Autodesk Inventor part; units mm, degrees
(part 5 of 6)
  line L796 (-0.8981, -221.2353) -> (-1.2073, -221.1704) construction
  line L797 (-1.2073, -221.1704) -> (-1.274, -221.1564) construction
  line L798 (-1.274, -221.1564) -> (-1.3926, -221.1187) construction
  line L799 (-1.3926, -221.1187) -> (-1.5231, -221.0797) construction
  line L800 (5.0298, -224.2577) -> (4.9095, -225.6862) construction
  spline S57 degree 3 poles (5.254, -220.972) (5.1998, -222.0685) (5.122, -223.1637) (5.0298, -224.2577) (4.9095, -225.6862) (4.7534, -227.1125) (4.551, -228.5318) (4.3466, -229.9645) (4.0271, -231.4371) (4.0386, -232.8878) (4.0462, -233.8475) (5.2747, -233.8855) (5.6006, -233.0992) (6.3871, -231.2018) (6.5459, -228.982) (6.7906, -226.9594) (7.0368, -224.9246) (7.1993, -222.8825) (7.2738, -220.8341) (7.2885, -220.4289) (7.3025, -220.0233) (7.3103, -219.6178) knots 5.14687 5.14687 5.14687 5.14687 6 6 6 7 7 7 8 8 8 9 9 9 10 10 10 11 11 11 11.773986 11.773986 11.773986 11.773986
  line L801 (5.254, -220.972) -> (5.1998, -222.0685) construction
  line L802 (5.1998, -222.0685) -> (5.122, -223.1637) construction
  line L803 (5.122, -223.1637) -> (5.0298, -224.2577) construction
  line L804 (4.9095, -225.6862) -> (4.7534, -227.1125) construction
  line L805 (4.7534, -227.1125) -> (4.551, -228.5318) construction
  line L806 (4.551, -228.5318) -> (4.3466, -229.9645) construction
  line L807 (4.3466, -229.9645) -> (4.0271, -231.4371) construction
  line L808 (4.0271, -231.4371) -> (4.0386, -232.8878) construction
  line L809 (4.0386, -232.8878) -> (4.0462, -233.8475) construction
  line L810 (4.0462, -233.8475) -> (5.2747, -233.8855) construction
  line L811 (5.2747, -233.8855) -> (5.6006, -233.0992) construction
  line L812 (5.6006, -233.0992) -> (6.3871, -231.2018) construction
  line L813 (6.3871, -231.2018) -> (6.5459, -228.982) construction
  line L814 (6.5459, -228.982) -> (6.7906, -226.9594) construction
  line L815 (6.7906, -226.9594) -> (7.0368, -224.9246) construction
  line L816 (7.0368, -224.9246) -> (7.1993, -222.8825) construction
  line L817 (7.1993, -222.8825) -> (7.2738, -220.8341) construction
  line L818 (7.2738, -220.8341) -> (7.2885, -220.4289) construction
  line L819 (7.2885, -220.4289) -> (7.3025, -220.0233) construction
  line L820 (7.3025, -220.0233) -> (7.3103, -219.6178) construction
  line L821 (-2.0297, -225.1684) -> (-2.0388, -225.06) construction
  spline S58 degree 3 poles (-2.0297, -225.1684) (-2.0388, -225.06) (-2.0694, -224.9045) (-2.0732, -224.8323) knots 8.458233 8.458233 8.458233 8.458233 9 9 9 9
  line L822 (-2.0388, -225.06) -> (-2.0694, -224.9045) construction
  line L823 (-2.0694, -224.9045) -> (-2.0732, -224.8323) construction
  line L824 (-2.0856, -224.5997) -> (-2.0972, -224.3671) construction
  spline S59 degree 3 poles (-2.0732, -224.8323) (-2.0856, -224.5997) (-2.0972, -224.3671) (-2.109, -224.1346) knots 9 9 9 9 10 10 10 10
  line L825 (-2.0732, -224.8323) -> (-2.0856, -224.5997) construction
  line L826 (-2.0972, -224.3671) -> (-2.109, -224.1346) construction
  line L827 (-1.5231, -221.0797) -> (-1.328, -220.9404) construction
  spline S60 degree 3 poles (-1.5231, -221.0797) (-1.328, -220.9404) (-1.1366, -220.7956) (-0.9498, -220.6454) (-0.1242, -219.9816) (0.9816, -219.0458) (1.2926, -217.9913) (2.0159, -215.5393) (-1.1884, -215.1481) (-2.8267, -215.345) (-5.2805, -215.6397) (-7.7108, -216.8198) (-9.2996, -218.7397) (-9.8909, -219.4541) (-8.9514, -220.4463) (-8.2639, -219.7754) knots 21.261625 21.261625 21.261625 21.261625 22 22 22 23 23 23 24 24 24 25 25 25 26 26 26 26
  line L828 (-1.328, -220.9404) -> (-1.1366, -220.7956) construction
  line L829 (-1.1366, -220.7956) -> (-0.9498, -220.6454) construction
  line L830 (-0.9498, -220.6454) -> (-0.1242, -219.9816) construction
  line L831 (-0.1242, -219.9816) -> (0.9816, -219.0458) construction
  line L832 (0.9816, -219.0458) -> (1.2926, -217.9913) construction
  line L833 (1.2926, -217.9913) -> (2.0159, -215.5393) construction
  line L834 (2.0159, -215.5393) -> (-1.1884, -215.1481) construction
  line L835 (-1.1884, -215.1481) -> (-2.8267, -215.345) construction
  line L836 (-2.8267, -215.345) -> (-5.2805, -215.6397) construction
  line L837 (-5.2805, -215.6397) -> (-7.7108, -216.8198) construction
  line L838 (-7.7108, -216.8198) -> (-9.2996, -218.7397) construction
  line L839 (-9.2996, -218.7397) -> (-9.8909, -219.4541) construction
  line L840 (-9.8909, -219.4541) -> (-8.9514, -220.4463) construction
  line L841 (-8.9514, -220.4463) -> (-8.2639, -219.7754) construction
  line L842 (-2.1476, -223.2875) -> (-2.1533, -222.8634) construction
  spline S61 degree 3 poles (-2.109, -224.1346) (-2.1305, -223.7108) (-2.1476, -223.2875) (-2.1533, -222.8634) knots 10 10 10 10 10.82684 10.82684 10.82684 10.82684
  line L843 (-2.109, -224.1346) -> (-2.1305, -223.7108) construction
  line L844 (-2.1305, -223.7108) -> (-2.1476, -223.2875) construction
  line L845 (4.252, -221.2799) -> (5.254, -220.972) construction
  spline S62 degree 3 poles (2.1677, -216.0966) (0.6747, -217.2243) (0.7113, -219.4286) (2.2363, -220.5301) (3.1577, -221.1955) (4.252, -221.2799) (5.254, -220.972) knots 0 0 0 0 1 1 1 1.551759 1.551759 1.551759 1.551759
  line L846 (2.1677, -216.0966) -> (0.6747, -217.2243) construction
  line L847 (0.6747, -217.2243) -> (0.7113, -219.4286) construction
  line L848 (0.7113, -219.4286) -> (2.2363, -220.5301) construction
  line L849 (2.2363, -220.5301) -> (3.1577, -221.1955) construction
  line L850 (3.1577, -221.1955) -> (4.252, -221.2799) construction
  line L851 (7.3103, -219.6178) -> (7.3306, -219.5942) construction
  spline S63 degree 3 poles (7.3103, -219.6178) (7.3306, -219.5942) (7.3507, -219.5703) (7.3705, -219.5463) (7.9707, -218.8184) (8.5772, -217.7782) (7.9557, -216.8786) (7.3563, -216.011) (6.1286, -216.1196) (5.6288, -217.0177) (5.3108, -217.589) (5.2677, -218.349) (5.2721, -219.0878) knots 1.983848 1.983848 1.983848 1.983848 2 2 2 3 3 3 4 4 4 4.613609 4.613609 4.613609 4.613609
  line L852 (7.3306, -219.5942) -> (7.3507, -219.5703) construction
  line L853 (7.3507, -219.5703) -> (7.3705, -219.5463) construction
  line L854 (7.3705, -219.5463) -> (7.9707, -218.8184) construction
  line L855 (7.9707, -218.8184) -> (8.5772, -217.7782) construction
  line L856 (8.5772, -217.7782) -> (7.9557, -216.8786) construction
  line L857 (7.9557, -216.8786) -> (7.3563, -216.011) construction
  line L858 (7.3563, -216.011) -> (6.1286, -216.1196) construction
  line L859 (6.1286, -216.1196) -> (5.6288, -217.0177) construction
  line L860 (5.6288, -217.0177) -> (5.3108, -217.589) construction
  line L861 (5.3108, -217.589) -> (5.2677, -218.349) construction
  line L862 (5.2677, -218.349) -> (5.2721, -219.0878) construction
  line L863 (5.2721, -219.0878) -> (5.1898, -219.1386) construction
  spline S64 degree 3 poles (5.2721, -219.0878) (5.1898, -219.1386) (5.1044, -219.1847) (5.0157, -219.2254) (4.3643, -219.5238) (3.4605, -219.4778) (2.9536, -218.9221) (2.5045, -218.4298) (2.5751, -217.6746) (3.0552, -217.2469) (3.6655, -216.7032) (2.837, -215.591) (2.1677, -216.0966) knots 16.74527 16.74527 16.74527 16.74527 17 17 17 18 18 18 19 19 19 20 20 20 20
  line L864 (5.1898, -219.1386) -> (5.1044, -219.1847) construction
  line L865 (5.1044, -219.1847) -> (5.0157, -219.2254) construction
  line L866 (5.0157, -219.2254) -> (4.3643, -219.5238) construction
  line L867 (4.3643, -219.5238) -> (3.4605, -219.4778) construction
  line L868 (3.4605, -219.4778) -> (2.9536, -218.9221) construction
  line L869 (2.9536, -218.9221) -> (2.5045, -218.4298) construction
  line L870 (2.5045, -218.4298) -> (2.5751, -217.6746) construction
  line L871 (2.5751, -217.6746) -> (3.0552, -217.2469) construction
  line L872 (3.0552, -217.2469) -> (3.6655, -216.7032) construction
  line L873 (3.6655, -216.7032) -> (2.837, -215.591) construction
  line L874 (2.837, -215.591) -> (2.1677, -216.0966) construction
  circle A5 centre (6.8365, -217.7782) radius 0.6286
  line L875 (-1.4966, -218.9144) -> (-2.1126, -219.3576) construction
  spline S65 degree 3 poles (-8.2639, -219.7754) (-6.7861, -218.3333) (-5.0043, -217.3238) (-2.9422, -217.0238) (-2.3715, -216.9407) (-0.7769, -216.6798) (-0.3673, -217.2886) (-0.0416, -217.7728) (-1.4966, -218.9144) (-2.1126, -219.3576) knots 0 0 0 0 1 1 1 2 2 2 2.88117 2.88117 2.88117 2.88117
  line L876 (-8.2639, -219.7754) -> (-6.7861, -218.3333) construction
  line L877 (-6.7861, -218.3333) -> (-5.0043, -217.3238) construction
  line L878 (-5.0043, -217.3238) -> (-2.9422, -217.0238) construction
  line L879 (-2.9422, -217.0238) -> (-2.3715, -216.9407) construction
  line L880 (-2.3715, -216.9407) -> (-0.7769, -216.6798) construction
  line L881 (-0.7769, -216.6798) -> (-0.3673, -217.2886) construction
  line L882 (-0.3673, -217.2886) -> (-0.0416, -217.7728) construction
  line L883 (-0.0416, -217.7728) -> (-1.4966, -218.9144) construction
  point P0 (0, 0)
  point P1 (-89.8672, -198.2095)
  point P2 (-69.9742, -200.3683)
  point P3 (-75.8668, -170.3202)
  point P4 (-42.8129, -214.4515)
  point P5 (-41.2254, -216.039)
  point P6 (-53.6547, -194.1688)
  point P7 (-90.9293, -176.9978)
  point P8 (-2.0909, -219.5286)
  constraints: 6 centre point, 180 other
extrude "Extrusion5" add sketch "Sketch6" against normal up to surface (3.175 mm away)
sketch "Sketch7" plane through (0, 3.175, 0) normal (0, 1, 0) x (1, 0, 0)
  circle A0 centre (16.8645, 29.5775) radius 1.25 projected
  circle A1 centre (-15.1355, 29.5775) radius 1.25 projected
  circle A2 centre (-15.1355, 61.5775) radius 1.25 projected
  circle A3 centre (16.8645, 61.5775) radius 1.25 projected
  arc A4 (15.8645, 52.5775) -> (15.8645, 54.5775) centre (15.8645, 53.5775) ccw projected
  line L0 (15.8645, 52.5775) -> (-23.218, 52.5775) projected
  arc A5 (-23.218, 52.5775) -> (-23.218, 50.5775) centre (-23.218, 51.5775) ccw projected
  line L1 (-23.218, 50.5775) -> (15.8645, 50.5775) projected
  arc A6 (15.8645, 48.5775) -> (15.8645, 50.5775) centre (15.8645, 49.5775) ccw projected
  line L2 (15.8645, 48.5775) -> (-23.218, 48.5775) projected
  arc A7 (-23.218, 48.5775) -> (-23.218, 46.5775) centre (-23.218, 47.5775) ccw projected
  line L3 (-23.218, 46.5775) -> (15.8645, 46.5775) projected
  arc A8 (15.8645, 44.5775) -> (15.8645, 46.5775) centre (15.8645, 45.5775) ccw projected
  line L4 (15.8645, 44.5775) -> (-23.218, 44.5775) projected
  arc A9 (-23.218, 44.5775) -> (-23.218, 42.5775) centre (-23.218, 43.5775) ccw projected
  line L5 (-23.218, 42.5775) -> (15.8645, 42.5775) projected
  arc A10 (15.8645, 40.5775) -> (15.8645, 42.5775) centre (15.8645, 41.5775) ccw projected
  line L6 (15.8645, 40.5775) -> (-23.218, 40.5775) projected
  arc A11 (-23.218, 40.5775) -> (-23.218, 38.5775) centre (-23.218, 39.5775) ccw projected
  line L7 (-23.218, 38.5775) -> (15.8645, 38.5775) projected
  arc A12 (15.8645, 36.5775) -> (15.8645, 38.5775) centre (15.8645, 37.5775) ccw projected
  line L8 (15.8645, 36.5775) -> (-23.218, 36.5775) projected
  arc A13 (-23.218, 36.5775) -> (-23.218, 34.5775) centre (-23.218, 35.5775) ccw projected
  line L9 (-23.218, 34.5775) -> (15.8645, 34.5775) projected
  arc A14 (15.8645, 32.5775) -> (15.8645, 34.5775) centre (15.8645, 33.5775) ccw projected
  line L10 (15.8645, 32.5775) -> (-21.0398, 32.5775) projected
  arc A15 (-21.0398, 32.5775) -> (-26.4124, 32.0925) centre (-21.0398, 2.5775) ccw projected
  arc A16 (-31.785, 31.6075) -> (-26.4124, 32.0925) centre (-31.785, 61.6075) ccw projected
  line L11 (-31.785, 31.6075) -> (-33.743, 31.6075) projected
  arc A17 (-33.743, 31.6075) -> (-40.093, 25.2575) centre (-33.743, 25.2575) ccw projected
  line L12 (-40.093, 25.2575) -> (-40.093, 19.225) projected
  arc A18 (-40.093, 19.225) -> (-38.5055, 17.6375) centre (-38.5055, 19.225) ccw projected
  line L13 (-38.5055, 17.6375) -> (36.4245, 17.6375) projected
  arc A19 (36.4245, 17.6375) -> (38.012, 19.225) centre (36.4245, 19.225) ccw projected
  line L14 (38.012, 19.225) -> (38.012, 71.9264) projected
  arc A20 (38.012, 71.9264) -> (36.4245, 73.5139) centre (36.4245, 71.9264) ccw projected
  line L15 (36.4245, 73.5139) -> (-37.8705, 73.5139) projected
  arc A21 (-37.8705, 73.5139) -> (-39.458, 71.9264) centre (-37.8705, 71.9264) ccw projected
  line L16 (-39.458, 71.9264) -> (-39.458, 65.8975) projected
  arc A22 (-39.458, 65.8975) -> (-33.108, 59.5475) centre (-33.108, 65.8975) ccw projected
  line L17 (-33.108, 59.5475) -> (-31.785, 59.5475) projected
  arc A23 (-26.4124, 59.0625) -> (-31.785, 59.5475) centre (-31.785, 29.5475) ccw projected
  arc A24 (-26.4124, 59.0625) -> (-21.0398, 58.5775) centre (-21.0398, 88.5775) ccw projected
  line L18 (-21.0398, 58.5775) -> (15.8645, 58.5775) projected
  arc A25 (15.8645, 56.5775) -> (15.8645, 58.5775) centre (15.8645, 57.5775) ccw projected
  line L19 (15.8645, 56.5775) -> (-23.218, 56.5775) projected
  arc A26 (-23.218, 56.5775) -> (-23.218, 54.5775) centre (-23.218, 55.5775) ccw projected
  line L20 (-23.218, 54.5775) -> (15.8645, 54.5775) projected
  circle A27 centre (16.6963, -6.4758) radius 1.25 projected
  circle A28 centre (-15.3037, -38.4758) radius 1.25 projected
  circle A29 centre (-15.3037, -6.4758) radius 1.25 projected
  circle A30 centre (16.6963, -38.4758) radius 1.25 projected
  line L21 (-33.2762, -8.5058) -> (-31.9532, -8.5058) projected
  arc A31 (-26.5806, -8.9908) -> (-31.9532, -8.5058) centre (-31.9532, -38.5058) ccw projected
  arc A32 (-26.5806, -8.9908) -> (-21.208, -9.4758) centre (-21.208, 20.5242) ccw projected
  line L22 (-21.208, -9.4758) -> (15.6963, -9.4758) projected
  arc A33 (15.6963, -11.4758) -> (15.6963, -9.4758) centre (15.6963, -10.4758) ccw projected
  line L23 (15.6963, -11.4758) -> (-23.3862, -11.4758) projected
  arc A34 (-23.3862, -11.4758) -> (-23.3862, -13.4758) centre (-23.3862, -12.4758) ccw projected
  line L24 (-23.3862, -13.4758) -> (15.6963, -13.4758) projected
  arc A35 (15.6963, -15.4758) -> (15.6963, -13.4758) centre (15.6963, -14.4758) ccw projected
  line L25 (15.6963, -15.4758) -> (-23.3862, -15.4758) projected
  arc A36 (-23.3862, -15.4758) -> (-23.3862, -17.4758) centre (-23.3862, -16.4758) ccw projected
  line L26 (-23.3862, -17.4758) -> (15.6963, -17.4758) projected
  arc A37 (15.6963, -19.4758) -> (15.6963, -17.4758) centre (15.6963, -18.4758) ccw projected
  line L27 (15.6963, -19.4758) -> (-23.3862, -19.4758) projected
  arc A38 (-23.3862, -19.4758) -> (-23.3862, -21.4758) centre (-23.3862, -20.4758) ccw projected
  line L28 (-23.3862, -21.4758) -> (15.6963, -21.4758) projected
  arc A39 (15.6963, -23.4758) -> (15.6963, -21.4758) centre (15.6963, -22.4758) ccw projected
  line L29 (15.6963, -23.4758) -> (-23.3862, -23.4758) projected
  arc A40 (-23.3862, -23.4758) -> (-23.3862, -25.4758) centre (-23.3862, -24.4758) ccw projected
  line L30 (-23.3862, -25.4758) -> (15.6963, -25.4758) projected
  arc A41 (15.6963, -27.4758) -> (15.6963, -25.4758) centre (15.6963, -26.4758) ccw projected
  line L31 (15.6963, -27.4758) -> (-23.3862, -27.4758) projected
  arc A42 (-23.3862, -27.4758) -> (-23.3862, -29.4758) centre (-23.3862, -28.4758) ccw projected
  line L32 (-23.3862, -29.4758) -> (15.6963, -29.4758) projected
  arc A43 (15.6963, -31.4758) -> (15.6963, -29.4758) centre (15.6963, -30.4758) ccw projected
  line L33 (15.6963, -31.4758) -> (-23.3862, -31.4758) projected
  arc A44 (-23.3862, -31.4758) -> (-23.3862, -33.4758) centre (-23.3862, -32.4758) ccw projected
  line L34 (-23.3862, -33.4758) -> (15.6963, -33.4758) projected
  arc A45 (15.6963, -35.4758) -> (15.6963, -33.4758) centre (15.6963, -34.4758) ccw projected
  line L35 (15.6963, -35.4758) -> (-21.208, -35.4758) projected
  arc A46 (-21.208, -35.4758) -> (-26.5806, -35.9608) centre (-21.208, -65.4758) ccw projected
  arc A47 (-31.9532, -36.4458) -> (-26.5806, -35.9608) centre (-31.9532, -6.4458) ccw projected
  line L36 (-31.9532, -36.4458) -> (-33.9112, -36.4458) projected
  arc A48 (-33.9112, -36.4458) -> (-40.2612, -42.7958) centre (-33.9112, -42.7958) ccw projected
  line L37 (-40.2612, -42.7958) -> (-40.2612, -48.8283) projected
  arc A49 (-40.2612, -48.8283) -> (-38.6737, -50.4158) centre (-38.6737, -48.8283) ccw projected
  line L38 (-38.6737, -50.4158) -> (36.2563, -50.4158) projected
  arc A50 (36.2563, -50.4158) -> (37.8438, -48.8283) centre (36.2563, -48.8283) ccw projected
  line L39 (37.8438, -48.8283) -> (37.8438, 3.8731) projected
  arc A51 (37.8438, 3.8731) -> (36.2563, 5.4606) centre (36.2563, 3.8731) ccw projected
  line L40 (36.2563, 5.4606) -> (-38.0387, 5.4606) projected
  arc A52 (-38.0387, 5.4606) -> (-39.6262, 3.8731) centre (-38.0387, 3.8731) ccw projected
  line L41 (-39.6262, 3.8731) -> (-39.6262, -2.1558) projected
  arc A53 (-39.6262, -2.1558) -> (-33.2762, -8.5058) centre (-33.2762, -2.1558) ccw projected
  line L42 (48.3343, -57.616) -> (-46.3157, -57.616) projected
  arc A54 (-49.4907, -54.441) -> (-46.3157, -57.616) centre (-46.3157, -54.441) ccw projected
  line L43 (-49.4907, -54.441) -> (-49.4907, 82.209) projected
  arc A55 (-46.3157, 85.384) -> (-49.4907, 82.209) centre (-46.3157, 82.209) ccw projected
  line L44 (-46.3157, 85.384) -> (48.3343, 85.384) projected
  arc A56 (51.5093, 82.209) -> (48.3343, 85.384) centre (48.3343, 82.209) ccw projected
  line L45 (51.5093, 82.209) -> (51.5093, -54.441) projected
  arc A57 (48.3343, -57.616) -> (51.5093, -54.441) centre (48.3343, -54.441) ccw projected
  arc A58 (13.6478, -234.0466) -> (14.6363, -233.1974) centre (13.6478, -233.0466) ccw projected
  line L46 (13.6478, -234.0466) -> (-11.6292, -234.0466) projected
  arc A59 (-12.6177, -233.1974) -> (-11.6292, -234.0466) centre (-11.6292, -233.0466) ccw projected
  arc A60 (-12.9607, -228.674) -> (-12.6177, -233.1974) centre (17.0393, -228.674) ccw projected
  line L47 (-12.9607, -228.674) -> (-12.9607, -220.366) projected
  line L48 (-6.6107, -214.016) -> (8.6293, -214.016) projected
  line L49 (14.9793, -220.366) -> (14.9793, -228.674) projected
  arc A61 (14.6363, -233.1974) -> (14.9793, -228.674) centre (-15.0207, -228.674) ccw projected
  line L50 (6.0093, -246.3235) -> (6.0093, -276.3235) projected
  arc A62 (4.0093, -276.3235) -> (6.0093, -276.3235) centre (5.0093, -276.3235) ccw projected
  line L51 (4.0093, -276.3235) -> (4.0093, -245.3235) projected
  line L52 (4.0093, -245.3235) -> (5.0093, -245.3235) projected
  arc A63 (6.0093, -246.3235) -> (5.0093, -245.3235) centre (5.0093, -246.3235) ccw projected
  line L53 (8.0093, -276.3235) -> (8.0093, -246.3235) projected
  arc A64 (10.0093, -246.3235) -> (8.0093, -246.3235) centre (9.0093, -246.3235) ccw projected
  line L54 (10.0093, -246.3235) -> (10.0093, -276.3235) projected
  arc A65 (8.0093, -276.3235) -> (10.0093, -276.3235) centre (9.0093, -276.3235) ccw projected
  line L55 (0.0093, -276.3235) -> (0.0093, -246.3235) projected
  arc A66 (2.0093, -246.3235) -> (0.0093, -246.3235) centre (1.0093, -246.3235) ccw projected
  line L56 (2.0093, -246.3235) -> (2.0093, -276.3235) projected
  arc A67 (0.0093, -276.3235) -> (2.0093, -276.3235) centre (1.0093, -276.3235) ccw projected
  line L57 (-3.9907, -276.3235) -> (-3.9907, -246.3235) projected
  arc A68 (-1.9907, -246.3235) -> (-3.9907, -246.3235) centre (-2.9907, -246.3235) ccw projected
  line L58 (-1.9907, -246.3235) -> (-1.9907, -276.3235) projected
  arc A69 (-3.9907, -276.3235) -> (-1.9907, -276.3235) centre (-2.9907, -276.3235) ccw projected
  line L59 (-7.9907, -276.3235) -> (-7.9907, -246.3235) projected
  arc A70 (-5.9907, -246.3235) -> (-7.9907, -246.3235) centre (-6.9907, -246.3235) ccw projected
  line L60 (-5.9907, -246.3235) -> (-5.9907, -276.3235) projected
  arc A71 (-7.9907, -276.3235) -> (-5.9907, -276.3235) centre (-6.9907, -276.3235) ccw projected
  line L61 (-11.9907, -276.3235) -> (-11.9907, -246.3235) projected
  arc A72 (-9.9907, -246.3235) -> (-11.9907, -246.3235) centre (-10.9907, -246.3235) ccw projected
  line L62 (-9.9907, -246.3235) -> (-9.9907, -276.3235) projected
  arc A73 (-11.9907, -276.3235) -> (-9.9907, -276.3235) centre (-10.9907, -276.3235) ccw projected
  line L63 (12.0093, -276.3235) -> (12.0093, -246.3235) projected
  arc A74 (14.0093, -246.3235) -> (12.0093, -246.3235) centre (13.0093, -246.3235) ccw projected
  line L64 (14.0093, -246.3235) -> (14.0093, -276.3235) projected
  arc A75 (12.0093, -276.3235) -> (14.0093, -276.3235) centre (13.0093, -276.3235) ccw projected
  circle A76 centre (92.1343, 51.998) radius 2.5527 projected
  circle A77 centre (92.1343, 74.223) radius 2.5527 projected
  circle A78 centre (92.1343, 29.773) radius 2.5527 projected
  circle A79 centre (92.1343, -14.677) radius 2.5527 projected
  circle A80 centre (92.1343, -59.127) radius 2.5527 projected
  circle A81 centre (92.1343, -103.577) radius 2.5527 projected
  circle A82 centre (92.1343, -125.802) radius 2.5527 projected
  circle A83 centre (92.1343, -81.352) radius 2.5527 projected
  circle A84 centre (92.1343, -36.902) radius 2.5527 projected
  circle A85 centre (92.1343, 7.548) radius 2.5527 projected
  circle A86 centre (-90.1157, 51.998) radius 2.5527 projected
  circle A87 centre (-90.1157, 7.548) radius 2.5527 projected
  circle A88 centre (-90.1157, -36.902) radius 2.5527 projected
  circle A89 centre (-90.1157, -81.352) radius 2.5527 projected
  circle A90 centre (-90.1157, -125.802) radius 2.5527 projected
  circle A91 centre (-90.1157, -103.577) radius 2.5527 projected
  circle A92 centre (-90.1157, -59.127) radius 2.5527 projected
  circle A93 centre (-90.1157, -14.677) radius 2.5527 projected
  circle A94 centre (-90.1157, 29.773) radius 2.5527 projected
  circle A95 centre (-90.1157, 74.223) radius 2.5527 projected
  circle A96 centre (1.0093, 127.4103) radius 2.5527 projected
  circle A97 centre (66.2468, -142.6982) radius 2.0193 projected
  circle A98 centre (-64.2282, -31.5732) radius 2.0193 projected
  circle A99 centre (66.2468, 79.5518) radius 2.0193 projected
  circle A100 centre (66.2468, -31.5732) radius 2.0193 projected
  circle A101 centre (-64.2282, 79.5518) radius 2.0193 projected
  circle A102 centre (-64.2282, -142.6982) radius 2.0193 projected
  circle A103 centre (-4.4907, -86.566) radius 1.6 projected
  circle A104 centre (-24.9907, -156.566) radius 1.6 projected
  circle A105 centre (27.0093, -73.616) radius 1.6 projected
  circle A106 centre (59.0093, -120.616) radius 1.6 projected
  circle A107 centre (59.0093, -73.616) radius 1.6 projected
  circle A108 centre (27.0093, -120.616) radius 1.6 projected
  circle A109 centre (-45.4907, -86.566) radius 1.6 projected
  circle A110 centre (-14.9907, -277.3235) radius 1.25 projected
  circle A111 centre (17.0093, -245.3235) radius 1.25 projected
  circle A112 centre (-14.9907, -245.3235) radius 1.25 projected
  circle A113 centre (17.0093, -277.3235) radius 1.25 projected
  line L65 (-26.9307, -253.9347) -> (-26.9307, -296.8835) projected
  arc A114 (-26.9307, -296.8835) -> (-25.3432, -298.471) centre (-25.3432, -296.8835) ccw projected
  line L66 (-25.3432, -298.471) -> (27.3618, -298.471) projected
  arc A115 (27.3618, -298.471) -> (28.9493, -296.8835) centre (27.3618, -296.8835) ccw projected
  line L67 (28.9493, -296.8835) -> (28.9493, -253.9347) projected
  arc A116 (33.1552, -225.0046) -> (28.9493, -253.9347) centre (130.5493, -253.9347) ccw projected
  line L68 (70.3843, -155.8506) -> (89.4343, -144.852) projected
  line L69 (101.6593, -123.6777) -> (101.6593, 85.3463) projected
  arc A117 (101.6593, 85.3463) -> (88.4997, 104.1401) centre (81.6593, 85.3463) ccw projected
  line L70 (88.4997, 104.1401) -> (18.1103, 129.7598) projected
  arc A118 (18.1103, 129.7598) -> (-16.0917, 129.7598) centre (1.0093, 82.7751) ccw projected
  line L71 (-16.0917, 129.7598) -> (-86.4811, 104.1401) projected
  arc A119 (-86.4811, 104.1401) -> (-99.6407, 85.3463) centre (-79.6407, 85.3463) ccw projected
  line L72 (-99.6407, 85.3463) -> (-99.6407, -123.6777) projected
  line L73 (-87.4157, -144.852) -> (-68.3657, -155.8506) projected
  arc A120 (-26.9307, -253.9347) -> (-31.1366, -225.0046) centre (-128.5307, -253.9347) ccw projected
  circle A121 centre (-86.7529, -269.1865) radius 1.25 projected
  circle A122 centre (-54.7529, -269.1865) radius 1.25 projected
  circle A123 centre (-86.7529, -237.1865) radius 1.25 projected
  circle A124 centre (-54.7529, -237.1865) radius 1.25 projected
  line L74 (-44.4004, -216.039) -> (-97.1018, -216.039) projected
  arc A125 (-97.1018, -216.039) -> (-98.6893, -217.6265) centre (-97.1018, -217.6265) ccw projected
  line L75 (-98.6893, -217.6265) -> (-98.6893, -291.9215) projected
  arc A126 (-98.6893, -291.9215) -> (-97.1018, -293.509) centre (-97.1018, -291.9215) ccw projected
  line L76 (-97.1018, -293.509) -> (-91.0729, -293.509) projected
  arc A127 (-91.0729, -293.509) -> (-84.7229, -287.159) centre (-91.0729, -287.159) ccw projected
  line L77 (-84.7229, -287.159) -> (-84.7229, -285.836) projected
  arc A128 (-84.2379, -280.4634) -> (-84.7229, -285.836) centre (-54.7229, -285.836) ccw projected
  arc A129 (-84.2379, -280.4634) -> (-83.7529, -275.0908) centre (-113.7529, -275.0908) ccw projected
  line L78 (-83.7529, -275.0908) -> (-83.7529, -238.1865) projected
  arc A130 (-81.7529, -238.1865) -> (-83.7529, -238.1865) centre (-82.7529, -238.1865) ccw projected
  line L79 (-81.7529, -238.1865) -> (-81.7529, -277.269) projected
  arc A131 (-81.7529, -277.269) -> (-79.7529, -277.269) centre (-80.7529, -277.269) ccw projected
  line L80 (-79.7529, -277.269) -> (-79.7529, -238.1865) projected
  arc A132 (-77.7529, -238.1865) -> (-79.7529, -238.1865) centre (-78.7529, -238.1865) ccw projected
  line L81 (-77.7529, -238.1865) -> (-77.7529, -277.269) projected
  arc A133 (-77.7529, -277.269) -> (-75.7529, -277.269) centre (-76.7529, -277.269) ccw projected
  line L82 (-75.7529, -277.269) -> (-75.7529, -238.1865) projected
  arc A134 (-73.7529, -238.1865) -> (-75.7529, -238.1865) centre (-74.7529, -238.1865) ccw projected
  line L83 (-73.7529, -238.1865) -> (-73.7529, -277.269) projected
  arc A135 (-73.7529, -277.269) -> (-71.7529, -277.269) centre (-72.7529, -277.269) ccw projected
  line L84 (-71.7529, -277.269) -> (-71.7529, -238.1865) projected
  arc A136 (-69.7529, -238.1865) -> (-71.7529, -238.1865) centre (-70.7529, -238.1865) ccw projected
  line L85 (-69.7529, -238.1865) -> (-69.7529, -277.269) projected
  arc A137 (-69.7529, -277.269) -> (-67.7529, -277.269) centre (-68.7529, -277.269) ccw projected
  line L86 (-67.7529, -277.269) -> (-67.7529, -238.1865) projected
  arc A138 (-65.7529, -238.1865) -> (-67.7529, -238.1865) centre (-66.7529, -238.1865) ccw projected
  line L87 (-65.7529, -238.1865) -> (-65.7529, -277.269) projected
  arc A139 (-65.7529, -277.269) -> (-63.7529, -277.269) centre (-64.7529, -277.269) ccw projected
  line L88 (-63.7529, -277.269) -> (-63.7529, -238.1865) projected
  arc A140 (-61.7529, -238.1865) -> (-63.7529, -238.1865) centre (-62.7529, -238.1865) ccw projected
  line L89 (-61.7529, -238.1865) -> (-61.7529, -277.269) projected
  arc A141 (-61.7529, -277.269) -> (-59.7529, -277.269) centre (-60.7529, -277.269) ccw projected
  line L90 (-59.7529, -277.269) -> (-59.7529, -238.1865) projected
  arc A142 (-57.7529, -238.1865) -> (-59.7529, -238.1865) centre (-58.7529, -238.1865) ccw projected
  line L91 (-57.7529, -238.1865) -> (-57.7529, -275.0908) projected
  arc A143 (-57.7529, -275.0908) -> (-57.2679, -280.4634) centre (-27.7529, -275.0908) ccw projected
  arc A144 (-56.7829, -285.836) -> (-57.2679, -280.4634) centre (-86.7829, -285.836) ccw projected
  line L92 (-56.7829, -285.836) -> (-56.7829, -287.794) projected
  arc A145 (-56.7829, -287.794) -> (-50.4329, -294.144) centre (-50.4329, -287.794) ccw projected
  line L93 (-50.4329, -294.144) -> (-44.4004, -294.144) projected
  arc A146 (-44.4004, -294.144) -> (-42.8129, -292.5565) centre (-44.4004, -292.5565) ccw projected
  line L94 (-42.8129, -292.5565) -> (-42.8129, -217.6265) projected
  arc A147 (-42.8129, -217.6265) -> (-44.4004, -216.039) centre (-44.4004, -217.6265) ccw projected
  circle A148 centre (88.5764, -269.6382) radius 1.25 projected
  circle A149 centre (56.5764, -269.6382) radius 1.25 projected
  circle A150 centre (56.5764, -237.6382) radius 1.25 projected
  circle A151 centre (88.5764, -237.6382) radius 1.25 projected
  arc A152 (46.2275, -216.4907) -> (44.64, -218.0782) centre (46.2275, -218.0782) ccw projected
  line L95 (44.64, -218.0782) -> (44.64, -292.3732) projected
  arc A153 (44.64, -292.3732) -> (46.2275, -293.9607) centre (46.2275, -292.3732) ccw projected
  line L96 (46.2275, -293.9607) -> (52.2564, -293.9607) projected
  arc A154 (52.2564, -293.9607) -> (58.6064, -287.6107) centre (52.2564, -287.6107) ccw projected
  line L97 (58.6064, -287.6107) -> (58.6064, -286.2877) projected
  arc A155 (59.0914, -280.9151) -> (58.6064, -286.2877) centre (88.6064, -286.2877) ccw projected
  arc A156 (59.0914, -280.9151) -> (59.5764, -275.5425) centre (29.5764, -275.5425) ccw projected
  line L98 (59.5764, -275.5425) -> (59.5764, -238.6382) projected
  arc A157 (61.5764, -238.6382) -> (59.5764, -238.6382) centre (60.5764, -238.6382) ccw projected
  line L99 (61.5764, -238.6382) -> (61.5764, -277.7207) projected
  arc A158 (61.5764, -277.7207) -> (63.5764, -277.7207) centre (62.5764, -277.7207) ccw projected
  line L100 (63.5764, -277.7207) -> (63.5764, -238.6382) projected
  arc A159 (65.5764, -238.6382) -> (63.5764, -238.6382) centre (64.5764, -238.6382) ccw projected
  line L101 (65.5764, -238.6382) -> (65.5764, -277.7207) projected
  arc A160 (65.5764, -277.7207) -> (67.5764, -277.7207) centre (66.5764, -277.7207) ccw projected
  line L102 (67.5764, -277.7207) -> (67.5764, -238.6382) projected
  arc A161 (69.5764, -238.6382) -> (67.5764, -238.6382) centre (68.5764, -238.6382) ccw projected
  line L103 (69.5764, -238.6382) -> (69.5764, -277.7207) projected
  arc A162 (69.5764, -277.7207) -> (71.5764, -277.7207) centre (70.5764, -277.7207) ccw projected
  line L104 (71.5764, -277.7207) -> (71.5764, -238.6382) projected
  arc A163 (73.5764, -238.6382) -> (71.5764, -238.6382) centre (72.5764, -238.6382) ccw projected
  line L105 (73.5764, -238.6382) -> (73.5764, -277.7207) projected
  arc A164 (73.5764, -277.7207) -> (75.5764, -277.7207) centre (74.5764, -277.7207) ccw projected
  line L106 (75.5764, -277.7207) -> (75.5764, -238.6382) projected
  arc A165 (77.5764, -238.6382) -> (75.5764, -238.6382) centre (76.5764, -238.6382) ccw projected
  line L107 (77.5764, -238.6382) -> (77.5764, -277.7207) projected
  arc A166 (77.5764, -277.7207) -> (79.5764, -277.7207) centre (78.5764, -277.7207) ccw projected
  line L108 (79.5764, -277.7207) -> (79.5764, -238.6382) projected
  arc A167 (81.5764, -238.6382) -> (79.5764, -238.6382) centre (80.5764, -238.6382) ccw projected
  line L109 (81.5764, -238.6382) -> (81.5764, -277.7207) projected
  arc A168 (81.5764, -277.7207) -> (83.5764, -277.7207) centre (82.5764, -277.7207) ccw projected
  line L110 (83.5764, -277.7207) -> (83.5764, -238.6382) projected
  arc A169 (85.5764, -238.6382) -> (83.5764, -238.6382) centre (84.5764, -238.6382) ccw projected
  line L111 (85.5764, -238.6382) -> (85.5764, -275.5425) projected
  arc A170 (85.5764, -275.5425) -> (86.0614, -280.9151) centre (115.5764, -275.5425) ccw projected
  arc A171 (86.5464, -286.2877) -> (86.0614, -280.9151) centre (56.5464, -286.2877) ccw projected
  line L112 (86.5464, -286.2877) -> (86.5464, -288.2457) projected
  arc A172 (86.5464, -288.2457) -> (92.8964, -294.5957) centre (92.8964, -288.2457) ccw projected
  line L113 (92.8964, -294.5957) -> (98.9289, -294.5957) projected
  arc A173 (98.9289, -294.5957) -> (100.5164, -293.0082) centre (98.9289, -293.0082) ccw projected
  line L114 (100.5164, -293.0082) -> (100.5164, -218.0782) projected
  arc A174 (100.5164, -218.0782) -> (98.9289, -216.4907) centre (98.9289, -218.0782) ccw projected
  line L115 (98.9289, -216.4907) -> (46.2275, -216.4907) projected
  circle A175 centre (94.9575, -171.3179) radius 1.9844 projected
  circle A176 centre (-64.2611, -168.0447) radius 0.8171 projected
  circle A177 centre (-80.9398, -196.4592) radius 0.6286 projected
  circle A178 centre (-61.0467, -198.6179) radius 0.6286 projected
  circle A179 centre (-82.0019, -175.2475) radius 0.6286 projected
  circle A180 centre (-42.049, -191.8933) radius 0.8171 projected
  circle A181 centre (6.8365, -217.7782) radius 0.6286 projected
  point P0 (0, 0)
  point P1 (31.027, 27.607)
  point P2 (31.027, 68.882)
  point P3 (-32.473, 68.882)
  point P4 (-32.473, 27.607)
  point P5 (-32.6412, -40.4463)
  point P6 (-32.6412, 0.8287)
  point P7 (30.8588, 0.8287)
  point P8 (30.8588, -40.4463)
  point P9 (-16.9612, -227.986)
  point P10 (24.3138, -227.986)
  point P11 (-16.9612, -291.486)
  point P12 (24.3138, -291.486)
  point P13 (39.2746, -199.7275)
  point P14 (-37.256, -199.7275)
  point P15 (-94.0574, -286.524)
  point P16 (-52.7824, -286.524)
  point P17 (-94.0574, -223.024)
  point P18 (-52.7824, -223.024)
  point P19 (49.2719, -286.9757)
  point P20 (90.5469, -286.9757)
  point P21 (90.5469, -223.4757)
  point P22 (49.2719, -223.4757)
  point P23 (79.7276, -173.2637)
  point P24 (90.8611, -179.8499)
  point P25 (96.3446, -176.2385)
  point P26 (90.9094, -174.8252)
  point P27 (82.6309, -166.8487)
  point P28 (80.5123, -169.3422)
  point P29 (54.8134, -176.6589)
  point P30 (71.2168, -175.5448)
  point P31 (71.4379, -191.0403)
  point P32 (71.3219, -190.1438)
  point P33 (71.2265, -188.2833)
  point P34 (71.1084, -184.8935)
  point P35 (72.7888, -180.137)
  point P36 (-71.746, -168.9859)
  point P37 (-66.3184, -172.1966)
  point P38 (-63.6452, -170.4361)
  point P39 (-66.2949, -169.7471)
  point P40 (-70.3306, -165.8586)
  point P41 (-71.3634, -167.0741)
  point P42 (-83.8916, -170.6411)
  point P43 (-75.895, -170.0979)
  point P44 (-75.7872, -177.652)
  point P45 (-75.8438, -177.215)
  point P46 (-75.8903, -176.308)
  point P47 (-75.9478, -174.6554)
  point P48 (-75.1286, -172.3366)
  point P49 (-86.6974, -197.1832)
  point P50 (-82.5223, -199.653)
  point P51 (-80.466, -198.2987)
  point P52 (-82.5042, -197.7687)
  point P53 (-85.6086, -194.7775)
  point P54 (-86.4031, -195.7126)
  point P55 (-96.0402, -198.4564)
  point P56 (-89.8889, -198.0386)
  point P57 (-89.806, -203.8494)
  point P58 (-89.8495, -203.5132)
  point P59 (-89.8853, -202.8155)
  point P60 (-89.9296, -201.5443)
  point P61 (-89.2994, -199.7606)
  point P62 (-66.8043, -199.3419)
  point P63 (-62.6293, -201.8117)
  point P64 (-60.573, -200.4574)
  point P65 (-62.6111, -199.9275)
  point P66 (-65.7156, -196.9363)
  point P67 (-66.5101, -197.8713)
  point P68 (-76.1471, -200.6151)
  point P69 (-69.9958, -200.1973)
  point P70 (-69.913, -206.0081)
  point P71 (-69.9564, -205.6719)
  point P72 (-69.9922, -204.9742)
  point P73 (-70.0365, -203.7031)
  point P74 (-69.4064, -201.9194)
  point P75 (-87.7595, -175.9715)
  point P76 (-83.5844, -178.4412)
  point P77 (-81.5281, -177.087)
  point P78 (-83.5663, -176.557)
  point P79 (-86.6707, -173.5658)
  point P80 (-87.4652, -174.5009)
  point P81 (-97.1023, -177.2446)
  point P82 (-90.951, -176.8268)
  point P83 (-90.8681, -182.6377)
  point P84 (-90.9116, -182.3015)
  point P85 (-90.9474, -181.6038)
  point P86 (-90.9917, -180.3326)
  point P87 (-90.3615, -178.5489)
  point P88 (-49.5338, -192.8345)
  point P89 (-44.1063, -196.0452)
  point P90 (-41.4331, -194.2847)
  point P91 (-44.0827, -193.5957)
  point P92 (-48.1185, -189.7072)
  point P93 (-49.1513, -190.9227)
  point P94 (-61.6795, -194.4897)
  point P95 (-53.6828, -193.9465)
  point P96 (-53.5751, -201.5006)
  point P97 (-53.6316, -201.0636)
  point P98 (-53.6781, -200.1566)
  point P99 (-53.7357, -198.504)
  point P100 (-52.9165, -196.1852)
  point P101 (1.0789, -218.5022)
  point P102 (5.254, -220.972)
  point P103 (7.3103, -219.6178)
  point P104 (5.2721, -219.0878)
  point P105 (2.1677, -216.0966)
  point P106 (1.3732, -217.0316)
  point P107 (-8.2639, -219.7754)
  point P108 (-2.1126, -219.3576)
  point P109 (-2.0297, -225.1684)
  point P110 (-2.0732, -224.8323)
  point P111 (-2.109, -224.1346)
  point P112 (-2.1533, -222.8634)
  point P113 (-1.5231, -221.0797)
  constraints: 119 other
sketch "Sketch3" plane through (0, 3.175, 0) normal (0, 1, 0) x (1, 0, 0)
  arc A0 (65.8152, -302.4137) -> (65.4071, -302.9558) centre (65.8573, -302.87) ccw
  arc A1 (64.1415, -304.8227) -> (65.4071, -302.9558) centre (63.8384, -303.2548) ccw
  arc A2 (62.361, -303.4383) -> (64.1415, -304.8227) centre (63.857, -303.3514) ccw
  arc A3 (62.361, -303.4383) -> (61.8352, -303.0421) centre (61.9299, -303.4633) ccw
  arc A4 (61.8352, -303.0421) -> (60.982, -303.2465) centre (68.6893, -333.536) ccw
  arc A5 (60.982, -303.2465) -> (60.6637, -303.8458) centre (61.095, -303.6906) ccw
  arc A6 (59.7058, -305.8876) -> (60.6637, -303.8458) centre (59.1611, -304.3864) ccw
  arc A7 (57.7306, -304.7988) -> (59.7058, -305.8876) centre (59.1946, -304.4789) ccw
  arc A8 (57.7306, -304.7988) -> (57.1493, -304.4897) centre (57.3087, -304.891) ccw
  arc A9 (57.1493, -304.4897) -> (56.3385, -304.8251) centre (68.6893, -333.536) ccw
  arc A10 (56.3385, -304.8251) -> (56.118, -305.4668) centre (56.5196, -305.2461) ccw
  arc A11 (55.4912, -307.6334) -> (56.118, -305.4668) centre (54.7184, -306.2358) ccw
  arc A12 (53.37, -306.8669) -> (55.4912, -307.6334) centre (54.766, -306.3219) ccw
  arc A13 (53.37, -306.8669) -> (52.7475, -306.6525) centre (52.9678, -307.024) ccw
  arc A14 (52.7475, -306.6525) -> (51.9992, -307.1106) centre (68.6893, -333.536) ccw
  arc A15 (51.9992, -307.1106) -> (51.8818, -307.7789) centre (52.2439, -307.4981) ccw
  arc A16 (51.6017, -310.0169) -> (51.8818, -307.7789) centre (50.6197, -308.7575) ccw
  arc A17 (49.3867, -309.5917) -> (51.6017, -310.0169) centre (50.6802, -308.8351) ccw
  arc A18 (49.3867, -309.5917) -> (48.7383, -309.4774) centre (49.0139, -309.8097) ccw
  arc A19 (48.7383, -309.4774) -> (48.0709, -310.0469) centre (68.6893, -333.536) ccw
  arc A20 (48.0709, -310.0469) -> (48.0594, -310.7253) centre (48.3732, -310.3913) ccw
  arc A21 (48.1328, -312.9795) -> (48.0594, -310.7253) centre (46.966, -311.8892) ccw
  arc A22 (45.8786, -312.9061) -> (48.1328, -312.9795) centre (47.0379, -311.9564) ccw
  arc A23 (45.8786, -312.9061) -> (45.2203, -312.8946) centre (45.5446, -313.1797) ccw
  arc A24 (45.2203, -312.8946) -> (44.6502, -313.5615) centre (68.6893, -333.536) ccw
  arc A25 (44.6502, -313.5615) -> (44.745, -314.2334) centre (45.0027, -313.8544) ccw
  arc A26 (45.1702, -316.4484) -> (44.745, -314.2334) centre (43.8471, -315.554) ccw
  arc A27 (42.9322, -316.7285) -> (45.1702, -316.4484) centre (43.9286, -315.6091) ccw
  arc A28 (42.9322, -316.7285) -> (42.2803, -316.8201) centre (42.6451, -317.051) ccw
  arc A29 (42.2803, -316.8201) -> (41.8215, -317.5679) centre (68.6893, -333.536) ccw
  arc A30 (41.8215, -317.5679) -> (42.0202, -318.2167) centre (42.2154, -317.8021) ccw
  arc A31 (42.7867, -320.3379) -> (42.0202, -318.2167) centre (41.34, -319.6616) ccw
  arc A32 (40.6201, -320.9647) -> (42.7867, -320.3379) centre (41.4291, -319.7032) ccw
  arc A33 (40.6201, -320.9647) -> (39.9905, -321.1571) centre (40.3869, -321.3282) ccw
  arc A34 (39.9905, -321.1571) -> (39.6543, -321.9676) centre (68.6893, -333.536) ccw
  arc A35 (39.6543, -321.9676) -> (39.9521, -322.5773) centre (40.08, -322.1372) ccw
  arc A36 (41.0409, -324.5525) -> (39.9521, -322.5773) centre (39.5063, -324.1108) ccw
  arc A37 (38.9991, -325.5104) -> (41.0409, -324.5525) centre (39.6008, -324.138) ccw
  arc A38 (38.9991, -325.5104) -> (38.4073, -325.799) centre (38.8257, -325.9059) ccw
  arc A39 (38.4073, -325.799) -> (38.2021, -326.6521) centre (68.6893, -333.536) ccw
  arc A40 (38.2021, -326.6521) -> (38.5916, -327.2077) centre (38.6491, -326.753) ccw
  arc A41 (39.976, -328.9882) -> (38.5916, -327.2077) centre (38.3911, -328.792) ccw
  arc A42 (38.1091, -330.2538) -> (39.976, -328.9882) centre (38.4888, -328.8041) ccw
  arc A43 (38.1091, -330.2538) -> (37.5698, -330.6314) centre (37.9997, -330.6715) ccw
  arc A44 (37.5698, -330.6314) -> (37.5005, -331.5061) centre (68.6893, -333.536) ccw
  arc A45 (37.5005, -331.5061) -> (37.9722, -331.9939) centre (37.9579, -331.5358) ccw
  arc A46 (39.6181, -333.536) -> (37.9722, -331.9939) centre (38.022, -333.5901) ccw
  arc A47 (37.9722, -335.078) -> (39.6181, -333.536) centre (38.1204, -333.5868) ccw
  arc A48 (37.9722, -335.078) -> (37.4986, -335.5353) centre (37.9295, -335.5077) ccw
  arc A49 (37.4986, -335.5353) -> (37.567, -336.41) centre (68.6893, -333.536) ccw
  arc A50 (37.567, -336.41) -> (38.1091, -336.8181) centre (38.0233, -336.3679) ccw
  arc A51 (39.976, -338.0837) -> (38.1091, -336.8181) centre (38.4081, -338.3868) ccw
  arc A52 (38.5916, -339.8642) -> (39.976, -338.0837) centre (38.5047, -338.3682) ccw
  arc A53 (38.5916, -339.8642) -> (38.1953, -340.39) centre (38.6166, -340.2953) ccw
  arc A54 (38.1953, -340.39) -> (38.3998, -341.2433) centre (68.6893, -333.536) ccw
  arc A55 (38.3998, -341.2433) -> (38.9991, -341.5615) centre (38.8439, -341.1302) ccw
  arc A56 (41.0409, -342.5194) -> (38.9991, -341.5615) centre (39.5397, -343.0641) ccw
  arc A57 (39.9521, -344.4946) -> (41.0409, -342.5194) centre (39.6322, -343.0306) ccw
  arc A58 (39.9521, -344.4946) -> (39.643, -345.0759) centre (40.0443, -344.9165) ccw
  arc A59 (39.643, -345.0759) -> (39.9784, -345.8867) centre (68.6893, -333.536) ccw
  arc A60 (39.9784, -345.8867) -> (40.6201, -346.1072) centre (40.3993, -345.7056) ccw
  arc A61 (42.7867, -346.734) -> (40.6201, -346.1072) centre (41.3891, -347.5068) ccw
  arc A62 (42.0202, -348.8552) -> (42.7867, -346.734) centre (41.4752, -347.4592) ccw
  arc A63 (42.0202, -348.8552) -> (41.8058, -349.4777) centre (42.1772, -349.2574) ccw
  arc A64 (41.8058, -349.4777) -> (42.2639, -350.226) centre (68.6893, -333.536) ccw
  arc A65 (42.2639, -350.226) -> (42.9322, -350.3435) centre (42.6514, -349.9813) ccw
  arc A66 (45.1702, -350.6236) -> (42.9322, -350.3435) centre (43.9108, -351.6055) ccw
  arc A67 (44.745, -352.8386) -> (45.1702, -350.6236) centre (43.9884, -351.545) ccw
  arc A68 (44.745, -352.8386) -> (44.6307, -353.4869) centre (44.963, -353.2113) ccw
  arc A69 (44.6307, -353.4869) -> (45.2002, -354.1544) centre (68.6893, -333.536) ccw
  arc A70 (45.2002, -354.1544) -> (45.8786, -354.1658) centre (45.5446, -353.852) ccw
  arc A71 (48.1328, -354.0924) -> (45.8786, -354.1658) centre (47.0425, -355.2592) ccw
  arc A72 (48.0594, -356.3466) -> (48.1328, -354.0924) centre (47.1097, -355.1874) ccw
  arc A73 (48.0594, -356.3466) -> (48.0479, -357.0049) centre (48.333, -356.6806) ccw
  arc A74 (48.0479, -357.0049) -> (48.7148, -357.575) centre (68.6893, -333.536) ccw
  arc A75 (48.7148, -357.575) -> (49.3867, -357.4802) centre (49.0077, -357.2225) ccw
  arc A76 (51.6017, -357.055) -> (49.3867, -357.4802) centre (50.7073, -358.3781) ccw
  arc A77 (51.8818, -359.293) -> (51.6017, -357.055) centre (50.7624, -358.2966) ccw
  arc A78 (51.8818, -359.293) -> (51.9733, -359.9449) centre (52.2043, -359.5801) ccw
  arc A79 (51.9733, -359.9449) -> (52.7212, -360.4038) centre (68.6893, -333.536) ccw
  arc A80 (52.7212, -360.4038) -> (53.37, -360.205) centre (52.9554, -360.0098) ccw
  arc A81 (55.4912, -359.4386) -> (53.37, -360.205) centre (54.8149, -360.8852) ccw
  arc A82 (56.118, -361.6052) -> (55.4912, -359.4386) centre (54.8565, -360.7961) ccw
  arc A83 (56.118, -361.6052) -> (56.3104, -362.2348) centre (56.4814, -361.8383) ccw
  arc A84 (56.3104, -362.2348) -> (57.1209, -362.5709) centre (68.6893, -333.536) ccw
  arc A85 (57.1209, -362.5709) -> (57.7306, -362.2731) centre (57.2905, -362.1452) ccw
  arc A86 (59.7058, -361.1843) -> (57.7306, -362.2731) centre (59.264, -362.7189) ccw
  arc A87 (60.6637, -363.2262) -> (59.7058, -361.1843) centre (59.2913, -362.6244) ccw
  arc A88 (60.6637, -363.2262) -> (60.9523, -363.8179) centre (61.0592, -363.3995) ccw
  arc A89 (60.9523, -363.8179) -> (61.8054, -364.0231) centre (68.6893, -333.536) ccw
  arc A90 (61.8054, -364.0231) -> (62.361, -363.6336) centre (61.9063, -363.5761) ccw
  arc A91 (64.1415, -362.2492) -> (62.361, -363.6336) centre (63.9453, -363.8341) ccw
  arc A92 (65.4071, -364.1161) -> (64.1415, -362.2492) centre (63.9574, -363.7365) ccw
  arc A93 (65.4071, -364.1161) -> (65.7847, -364.6554) centre (65.8248, -364.2255) ccw
  arc A94 (65.7847, -364.6554) -> (66.6594, -364.7247) centre (68.6893, -333.536) ccw
  arc A95 (66.6594, -364.7247) -> (67.1472, -364.253) centre (66.6891, -364.2673) ccw
  arc A96 (68.6893, -362.6071) -> (67.1472, -364.253) centre (68.7434, -364.2032) ccw
  arc A97 (70.2313, -364.253) -> (68.6893, -362.6071) centre (68.7401, -364.1049) ccw
  arc A98 (70.2313, -364.253) -> (70.6886, -364.7266) centre (70.661, -364.2957) ccw
  arc A99 (70.6886, -364.7266) -> (71.5633, -364.6582) centre (68.6893, -333.536) ccw
  arc A100 (71.5633, -364.6582) -> (71.9714, -364.1161) centre (71.5212, -364.2019) ccw
  arc A101 (73.237, -362.2492) -> (71.9714, -364.1161) centre (73.5401, -363.8171) ccw
  arc A102 (75.0175, -363.6336) -> (73.237, -362.2492) centre (73.5215, -363.7206) ccw
  arc A103 (75.0175, -363.6336) -> (75.5433, -364.0299) centre (75.4486, -363.6086) ccw
  arc A104 (75.5433, -364.0299) -> (76.3966, -363.8255) centre (68.6893, -333.536) ccw
  arc A105 (76.3966, -363.8255) -> (76.7148, -363.2262) centre (76.2835, -363.3813) ccw
  arc A106 (77.6727, -361.1843) -> (76.7148, -363.2262) centre (78.2174, -362.6855) ccw
  arc A107 (79.6479, -362.2731) -> (77.6727, -361.1843) centre (78.1839, -362.593) ccw
  arc A108 (79.6479, -362.2731) -> (80.2292, -362.5822) centre (80.0698, -362.1809) ccw
  arc A109 (80.2292, -362.5822) -> (81.04, -362.2469) centre (68.6893, -333.536) ccw
  arc A110 (81.04, -362.2469) -> (81.2605, -361.6052) centre (80.8589, -361.8259) ccw
  arc A111 (81.8873, -359.4386) -> (81.2605, -361.6052) centre (82.6601, -360.8361) ccw
  arc A112 (84.0085, -360.205) -> (81.8873, -359.4386) centre (82.6125, -360.75) ccw
  arc A113 (84.0085, -360.205) -> (84.631, -360.4194) centre (84.4107, -360.048) ccw
  arc A114 (84.631, -360.4194) -> (85.3793, -359.9613) centre (68.6893, -333.536) ccw
  arc A115 (85.3793, -359.9613) -> (85.4967, -359.293) centre (85.1346, -359.5738) ccw
  arc A116 (85.7769, -357.055) -> (85.4967, -359.293) centre (86.7588, -358.3144) ccw
  arc A117 (87.9918, -357.4802) -> (85.7769, -357.055) centre (86.6983, -358.2369) ccw
  arc A118 (87.9918, -357.4802) -> (88.6402, -357.5946) centre (88.3646, -357.2622) ccw
  arc A119 (88.6402, -357.5946) -> (89.3077, -357.0251) centre (68.6893, -333.536) ccw
  arc A120 (89.3077, -357.0251) -> (89.3191, -356.3466) centre (89.0053, -356.6806) ccw
  arc A121 (89.2457, -354.0924) -> (89.3191, -356.3466) centre (90.4125, -355.1827) ccw
  arc A122 (91.4999, -354.1658) -> (89.2457, -354.0924) centre (90.3407, -355.1155) ccw
  arc A123 (91.4999, -354.1658) -> (92.1582, -354.1773) centre (91.8339, -353.8922) ccw
  arc A124 (92.1582, -354.1773) -> (92.7283, -353.5104) centre (68.6893, -333.536) ccw
  arc A125 (92.7283, -353.5104) -> (92.6335, -352.8386) centre (92.3758, -353.2176) ccw
  arc A126 (92.2083, -350.6236) -> (92.6335, -352.8386) centre (93.5314, -351.5179) ccw
  arc A127 (94.4463, -350.3435) -> (92.2083, -350.6236) centre (93.4499, -351.4628) ccw
  arc A128 (94.4463, -350.3435) -> (95.0982, -350.2519) centre (94.7334, -350.0209) ccw
  arc A129 (95.0982, -350.2519) -> (95.557, -349.504) centre (68.6893, -333.536) ccw
  arc A130 (95.557, -349.504) -> (95.3583, -348.8552) centre (95.1631, -349.2698) ccw
  arc A131 (94.5918, -346.734) -> (95.3583, -348.8552) centre (96.0385, -347.4103) ccw
  arc A132 (96.7584, -346.1072) -> (94.5918, -346.734) centre (95.9494, -347.3687) ccw
  arc A133 (96.7584, -346.1072) -> (97.388, -345.9148) centre (96.9916, -345.7438) ccw
  arc A134 (97.388, -345.9148) -> (97.7242, -345.1043) centre (68.6893, -333.536) ccw
  arc A135 (97.7242, -345.1043) -> (97.4264, -344.4946) centre (97.2985, -344.9347) ccw
  arc A136 (96.3376, -342.5194) -> (97.4264, -344.4946) centre (97.8722, -342.9612) ccw
  arc A137 (98.3794, -341.5615) -> (96.3376, -342.5194) centre (97.7777, -342.934) ccw
  arc A138 (98.3794, -341.5615) -> (98.9712, -341.2729) centre (98.5528, -341.166) ccw
  arc A139 (98.9712, -341.2729) -> (99.1764, -340.4199) centre (68.6893, -333.536) ccw
  arc A140 (99.1764, -340.4199) -> (98.7869, -339.8642) centre (98.7294, -340.3189) ccw
  arc A141 (97.4025, -338.0837) -> (98.7869, -339.8642) centre (98.9874, -338.2799) ccw
  arc A142 (99.2694, -336.8181) -> (97.4025, -338.0837) centre (98.8897, -338.2678) ccw
  arc A143 (99.2694, -336.8181) -> (99.8087, -336.4405) centre (99.3788, -336.4004) ccw
  arc A144 (99.8087, -336.4405) -> (99.878, -335.5659) centre (68.6893, -333.536) ccw
  arc A145 (99.878, -335.5659) -> (99.4063, -335.078) centre (99.4206, -335.5361) ccw
  arc A146 (97.7604, -333.536) -> (99.4063, -335.078) centre (99.3565, -333.4818) ccw
  arc A147 (99.4063, -331.9939) -> (97.7604, -333.536) centre (99.2582, -333.4852) ccw
  arc A148 (99.4063, -331.9939) -> (99.8799, -331.5366) centre (99.449, -331.5642) ccw
  arc A149 (99.8799, -331.5366) -> (99.8115, -330.6619) centre (68.6893, -333.536) ccw
  arc A150 (99.8115, -330.6619) -> (99.2694, -330.2538) centre (99.3552, -330.704) ccw
  arc A151 (97.4025, -328.9882) -> (99.2694, -330.2538) centre (98.9704, -328.6851) ccw
  arc A152 (98.7869, -327.2077) -> (97.4025, -328.9882) centre (98.8739, -328.7038) ccw
  arc A153 (98.7869, -327.2077) -> (99.1832, -326.6819) centre (98.7619, -326.7766) ccw
  arc A154 (99.1832, -326.6819) -> (98.9788, -325.8287) centre (68.6893, -333.536) ccw
  arc A155 (98.9788, -325.8287) -> (98.3794, -325.5104) centre (98.5346, -325.9417) ccw
  arc A156 (96.3376, -324.5525) -> (98.3794, -325.5104) centre (97.8388, -324.0078) ccw
  arc A157 (97.4264, -322.5773) -> (96.3376, -324.5525) centre (97.7463, -324.0413) ccw
  arc A158 (97.4264, -322.5773) -> (97.7355, -321.996) centre (97.3342, -322.1554) ccw
  arc A159 (97.7355, -321.996) -> (97.4002, -321.1852) centre (68.6893, -333.536) ccw
  arc A160 (97.4002, -321.1852) -> (96.7584, -320.9647) centre (96.9792, -321.3663) ccw
  arc A161 (94.5918, -320.3379) -> (96.7584, -320.9647) centre (95.9894, -319.5651) ccw
  arc A162 (95.3583, -318.2167) -> (94.5918, -320.3379) centre (95.9033, -319.6127) ccw
  arc A163 (95.3583, -318.2167) -> (95.5727, -317.5942) centre (95.2013, -317.8145) ccw
  arc A164 (95.5727, -317.5942) -> (95.1146, -316.8459) centre (68.6893, -333.536) ccw
  arc A165 (95.1146, -316.8459) -> (94.4463, -316.7285) centre (94.7271, -317.0906) ccw
  arc A166 (92.2083, -316.4484) -> (94.4463, -316.7285) centre (93.4677, -315.4664) ccw
  arc A167 (92.6335, -314.2334) -> (92.2083, -316.4484) centre (93.3902, -315.5269) ccw
  arc A168 (92.6335, -314.2334) -> (92.7479, -313.585) centre (92.4155, -313.8606) ccw
  arc A169 (92.7479, -313.585) -> (92.1784, -312.9176) centre (68.6893, -333.536) ccw
  arc A170 (92.1784, -312.9176) -> (91.4999, -312.9061) centre (91.8339, -313.2199) ccw
  arc A171 (89.2457, -312.9795) -> (91.4999, -312.9061) centre (90.336, -311.8127) ccw
  arc A172 (89.3191, -310.7253) -> (89.2457, -312.9795) centre (90.2688, -311.8846) ccw
  arc A173 (89.3191, -310.7253) -> (89.3306, -310.0671) centre (89.0455, -310.3913) ccw
  arc A174 (89.3306, -310.0671) -> (88.6637, -309.4969) centre (68.6893, -333.536) ccw
  arc A175 (88.6637, -309.4969) -> (87.9918, -309.5917) centre (88.3708, -309.8494) ccw
  arc A176 (85.7769, -310.0169) -> (87.9918, -309.5917) centre (86.6712, -308.6938) ccw
  arc A177 (85.4967, -307.7789) -> (85.7769, -310.0169) centre (86.6161, -308.7753) ccw
  arc A178 (85.4967, -307.7789) -> (85.4052, -307.127) centre (85.1742, -307.4918) ccw
  arc A179 (85.4052, -307.127) -> (84.6573, -306.6682) centre (68.6893, -333.536) ccw
  arc A180 (84.6573, -306.6682) -> (84.0085, -306.8669) centre (84.4231, -307.0621) ccw
  arc A181 (81.8873, -307.6334) -> (84.0085, -306.8669) centre (82.5636, -306.1867) ccw
  arc A182 (81.2605, -305.4668) -> (81.8873, -307.6334) centre (82.522, -306.2758) ccw
  arc A183 (81.2605, -305.4668) -> (81.0681, -304.8372) centre (80.8971, -305.2337) ccw
  arc A184 (81.0681, -304.8372) -> (80.2576, -304.501) centre (68.6893, -333.536) ccw
  arc A185 (80.2576, -304.501) -> (79.6479, -304.7988) centre (80.088, -304.9268) ccw
  arc A186 (77.6727, -305.8876) -> (79.6479, -304.7988) centre (78.1145, -304.353) ccw
  arc A187 (76.7148, -303.8458) -> (77.6727, -305.8876) centre (78.0872, -304.4475) ccw
  arc A188 (76.7148, -303.8458) -> (76.4262, -303.254) centre (76.3193, -303.6724) ccw
  arc A189 (76.4262, -303.254) -> (75.5731, -303.0488) centre (68.6893, -333.536) ccw
  arc A190 (75.5731, -303.0488) -> (75.0175, -303.4383) centre (75.4722, -303.4958) ccw
  arc A191 (73.237, -304.8227) -> (75.0175, -303.4383) centre (73.4332, -303.2378) ccw
  arc A192 (71.9714, -302.9558) -> (73.237, -304.8227) centre (73.4211, -303.3355) ccw